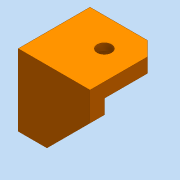
# Autodesk Inventor part: Frame2WayBlock
Saved by Autodesk Inventor 2016 (Build 200138000, 138)
## iProperties
Created: 2016-08-20
Part Number: Frame2WayBlock
Material: PLA Orange
Document SubType Name: Modeling
Designer: Sam
Density: 1 g/cm^3
Appearance: Generic
Author: Sam
Autodesk Inventor part; units mm, degrees
ref_plane "YZ Plane" through (0, 0, 0) normal (1, 0, 0) x (0, 1, 0)
ref_plane "XZ Plane" through (0, 0, 0) normal (0, 1, 0) x (-1, 0, 0)
ref_plane "XY Plane" through (0, 0, 0) normal (0, 0, 1) x (1, 0, 0)
sketch "Sketch1" plane through (0, 0, 0) normal (0, 1, 0) x (-1, 0, 0)
  line L0 (0, 0) -> (-20, 0)
  line L1 (-20, 0) -> (-20, -20)
  line L2 (-20, -20) -> (0, -20)
  line L3 (0, -20) -> (0, 0)
  dimension "d0" = 20
  dimension "d1" = 20
  constraints: 8 end point, 2 parallel, 1 horizontal, 1 perpendicular
  measures "d0" distance of L2.end L1.end
  measures "d1" distance of L1.end L0.end
extrude "Extrusion1" add sketch "Sketch1" along normal blind 4
sketch "Sketch2" plane through (0, 4, 0) normal (0, 1, 0) x (1, 0, 0)
  line L0 (0, 0) -> (20, 0)
  line L1 (20, 0) -> (20, 4)
  line L2 (20, 4) -> (4, 4)
  line L3 (0, 4) -> (0, 0)
  line L4 (0, 0) -> (4, 0)
  line L5 (4, 20) -> (0, 20)
  line L6 (0, 20) -> (0, 0)
  line L7 (4, 4) -> (4, 20)
  line L8 (0, 0) -> (20, 0) projected
  line L9 (0, 0) -> (20, 0)
  line L10 (0, 20) -> (0, 0) projected
  line L11 (0, 0) -> (0, 20)
  constraints: 20 end point, 4 parallel, 3 horizontal, 2 perpendicular, 1 vertical
extrude "Extrusion2" add sketch "Sketch2" along normal blind 16
hole "Hole2" at (12, 12, -4) direction (0, 0, 1) diameter 4 end through all
hole "Hole3" at (4, 12, -12) direction (-1, 0, 0) diameter 4 end through all
chamfer "Chamfer1" distance 12 angle 45 1 edges at (20, 2, -20)
chamfer "Chamfer2" distance 4 angle 45 1 edges at (20, 20, -2)
chamfer "Chamfer3" distance 4 angle 45 1 edges at (2, 20, -20)
sketch "Sketch3" plane through (20, 4, -4) normal (0, 0, -1) x (-1, 0, 0)
  line L0 (8, 12.0415) -> (11.5, 10.0207)
  line L1 (11.5, 10.0207) -> (11.5, 5.9793)
  line L2 (11.5, 5.9793) -> (8, 3.9585)
  line L3 (8, 3.9585) -> (4.5, 5.9793)
  line L4 (4.5, 5.9793) -> (4.5, 10.0207)
  line L5 (4.5, 10.0207) -> (8, 12.0415)
  point P0 (20, -4)
  point P1 (8, 8)
  dimension "d51" = 7
  constraints: 12 end point, 13 other
  measures "d51" distance between parallel lines of L1 L4
sketch "Sketch4" plane through (4, 4, -4) normal (1, 0, 0) x (0, 0, -1)
  line L0 (3.9585, 8) -> (5.9793, 11.5)
  line L1 (5.9793, 11.5) -> (10.0207, 11.5)
  line L2 (10.0207, 11.5) -> (12.0415, 8)
  line L3 (12.0415, 8) -> (10.0207, 4.5)
  line L4 (10.0207, 4.5) -> (5.9793, 4.5)
  line L5 (5.9793, 4.5) -> (3.9585, 8)
  point P0 (-4, -4)
  point P1 (8, 8)
  dimension "d52" = 7
  constraints: 12 end point, 13 other
  measures "d52" distance between parallel lines of L1 L4
extrude "Extrusion3" cut sketch "Sketch3" against normal blind 2
extrude "Extrusion4" cut sketch "Sketch4" against normal blind 2
body "Solid1"
